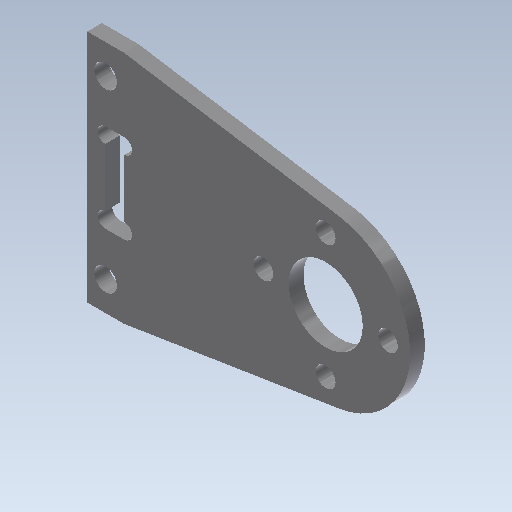
# Autodesk Inventor part: Shoulder_vertical_frame_02
Saved by Autodesk Inventor 2020.4 (Build 244396000, 396)
## iProperties
Created: 2016-05-05
Part Number: Shoulder_vertical_frame_02
Material: アルミニウム 2014-T4
Document SubType Name: Modeling
Designer: hiroaki
Density: 2.8 g/cm^3
Appearance: 滑らか - 淡い灰色
Mass: 3.06212 g
Surface Area: 18.1271 cm^2
Volume: 1.09361 cm^3
Description: A2017 T2
Author: hiroaki
Autodesk Inventor part; units mm, degrees
ref_plane "YZ Plane" through (0, 0, 0) normal (1, 0, 0) x (0, 1, 0)
ref_plane "XZ Plane" through (0, 0, 0) normal (0, 1, 0) x (-1, 0, 0)
ref_plane "XY Plane" through (0, 0, 0) normal (0, 0, 1) x (1, 0, 0)
sketch "スケッチ1" plane through (0, 0, 0) normal (0, 0, 1) x (1, 0, 0)
  circle A0 centre (0, 0) radius 10.5 construction
  circle A1 centre (0, 8.5) radius 1.35
  circle A2 centre (-8.5, 0) radius 1.35
  circle A3 centre (0, -8.5) radius 1.35
  circle A4 centre (8.5, 0) radius 1.35
  circle A5 centre (0, 0) radius 5.05
  line L0 (-30, 6) -> (-27.5, 6) construction
  line L1 (-27.5, 6) -> (-27.5, -6) construction
  line L2 (-27.5, -6) -> (-30, -6) construction
  line L3 (-30, -6) -> (-30, 6) construction
  line L4 (-27.45, 6.05) -> (-30.05, 6.05) construction
  line L5 (-30.05, 6.05) -> (-30.05, -6.05) construction
  line L6 (-30.05, -6.05) -> (-27.45, -6.05) construction
  line L7 (-27.45, -6.05) -> (-27.45, 6.05) construction
  circle A6 centre (-30.05, 5) radius 1.05 construction
  line L8 (-27.45, 6.05) -> (-30.05, 6.05)
  arc A7 (-30.05, 6.05) -> (-30.05, 3.95) centre (-30.05, 5) ccw
  line L9 (-30.05, 3.95) -> (-30.05, -3.95)
  line L10 (-28.75, 6.05) -> (-28.75, -6.05) construction
  line L11 (-30.05, 0) -> (-27.5, 0) construction
  arc A8 (-30.05, -3.95) -> (-30.05, -6.05) centre (-30.05, -5) ccw
  line L12 (-30.05, -6.05) -> (-27.45, -6.05)
  line L13 (-27.45, 3.95) -> (-27.45, -3.95)
  arc A9 (-27.45, 3.95) -> (-27.45, 6.05) centre (-27.45, 5) ccw
  arc A10 (-27.45, -6.05) -> (-27.45, -3.95) centre (-27.45, -5) ccw
  circle A11 centre (-30, 12) radius 1.55
  circle A12 centre (-30, -12) radius 1.55
  line L14 (-32.5, 16) -> (-27.5, 16)
  line L15 (-32.5, -16) -> (-27.5, -16)
  arc A13 (1.7994, -11.3584) -> (1.7994, 11.3584) centre (0, 0) ccw
  line L16 (-32.5, 16) -> (-32.5, -16)
  line L17 (-27.5, 16) -> (1.7994, 11.3584)
  line L18 (1.7994, -11.3584) -> (-27.5, -16)
  point P0 (-28.775, 0)
  dimension "d29" = 2.1
  dimension "d0" = 21
  dimension "d3" = 8.5
  dimension "d4" = 2.7
  dimension "d7" = 360
  dimension "d9" = 10.1
  dimension "d10" = 2.5
  dimension "d30" = 0.05
  dimension "d31" = 6
  dimension "d33" = 3.1
  dimension "d43" = 1
  dimension "d57" = 32
  dimension "d61" = 32.5
  dimension "d62" = 5
  dimension "d63" = 2.5
  dimension "d65" = 10
  constraints: 38 end point, 13 centre point, 10 point on circle, 5 coincident, 5 midpoint, 5 parallel, 5 symmetric about line, 5 tangent, 4 perpendicular, 4 vertical alignment, 3 horizontal, 2 collinear, 2 equal radius, 2 vertical, 1 horizontal alignment, 1 point on line, 16 other
  measures "d0" diameter of A0
  measures "d3" distance of point (0, 0) A1.centre
  measures "d4" diameter of A1
  measures "d9" diameter of A5
  measures "d10" distance of L0.start L0.end
  measures "d30" distance between parallel lines of L4 L0
  measures "d31" distance from line of L0 A11.centre
  measures "d33" diameter of A11
  measures "d43" radial gap between concentric circles of A13 A0
  measures "d57" distance of L15.start L14.start
  measures "d61" distance from line of point (0, 0) L16
  measures "d62" distance of L14.start L14.end
  measures "d63" horizontal distance of L14.start A11.centre
  measures "d65" distance between parallel lines of L14 L0
extrude "押し出し1" add sketch "スケッチ1" along normal blind 2
equation "\"d23\" = 7"
